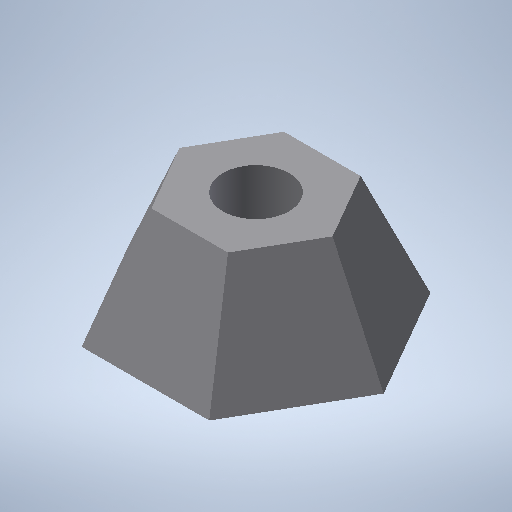
# Autodesk Inventor part: ai_param_dsdm_part1
Saved by Autodesk Inventor 2025 (Build 290162000, 162)
## iProperties
Shininess: 64.0
Length Units: 11269
Angle Units: 11279
Time Units: 11290
Mass Units: 11283
Length Display Precision: 3
Angle Display Precision: 2
Created: 2003-05-21
Part Number: ai_param_dsdm_part1
Document SubType Name: Modeling
Designer: vjcs
Density: 1 g/cm^3
Material: Generic
Appearance: Default
Density: 0.0
Volumn: 0.0
Area: 0.0
PropertySet Name: Model Information
Control State: 0
Master: False
Checked Out: False
Author: vjcs
Autodesk Inventor part; units mm, degrees
ref_plane "YZ Plane" through (0, 0, 0) normal (1, 0, 0) x (0, 1, 0)
ref_plane "XZ Plane" through (0, 0, 0) normal (0, 1, 0) x (-1, 0, 0)
sketch "Sketch3" plane through (0, 0, 0) normal (0, 0, 1) x (1, 0, 0)
  line L0 (28.8675, 50) -> (57.735, 0)
  line L1 (57.735, 0) -> (28.8675, -50)
  line L2 (28.8675, -50) -> (-28.8675, -50)
  line L3 (-28.8675, -50) -> (-57.735, 0)
  line L4 (-57.735, 0) -> (-28.8675, 50)
  line L5 (-28.8675, 50) -> (28.8675, 50)
  point P0 (0, 0)
  point P1 (0, 50)
  dimension "DS_HEX_R1" = 50
  constraints: 12 end point, 1 midpoint, 12 other
  measures "DS_HEX_R1" distance from line of L5 point (0, 0)
ref_plane "Work Plane1" through (0, 0, 50) normal (0, 0, 1) x (1, 0, 0)
sketch "Sketch4" plane through (0, 0, 50) normal (0, 0, 1) x (1, 0, 0)
  line L0 (17.3205, 30) -> (34.641, 0)
  line L1 (34.641, 0) -> (17.3205, -30)
  line L2 (17.3205, -30) -> (-17.3205, -30)
  line L3 (-17.3205, -30) -> (-34.641, 0)
  line L4 (-34.641, 0) -> (-17.3205, 30)
  line L5 (-17.3205, 30) -> (17.3205, 30)
  point P0 (0, 0)
  point P1 (0, 0)
  point P2 (0, 30)
  dimension "d16" = 0
  dimension "DS_HEX_R2" = 30
  constraints: 12 end point, 1 coincident, 1 midpoint, 12 other
  measures "DS_HEX_R2" distance from line of L5 point (0, 0)
loft "Loft1" add profiles "Sketch3", "Sketch4"
sketch "Sketch6" plane through (0, 0, 0) normal (0, 0, 1) x (1, 0, 0)
  point P0 (0, 0)
  constraints: 1 other
hole "Hole3" at (0, 0, 0) direction (0, 0, 1) diameter 30 end through all
body "Solid1"
